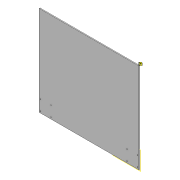
# Autodesk Inventor part: voetensteun
Saved by Autodesk Inventor 2020.3 (Build 243373000, 373)
## iProperties
Created: 2020-09-30
Part Number: voetensteun
Material: Generic
Document SubType Name: Sheet Metal
Designer: Svend
Density: 1 g/cm^3
Appearance: Default
Sheet Metal Rule: Default
Author: Svend
Autodesk Inventor part; units mm, degrees
ref_plane "YZ Plane" through (0, 0, 0) normal (1, 0, 0) x (0, 1, 0)
ref_plane "XZ Plane" through (0, 0, 0) normal (0, 1, 0) x (-1, 0, 0)
ref_plane "XY Plane" through (0, 0, 0) normal (0, 0, 1) x (1, 0, 0)
ref_plane "Work Plane1" through (0, 10, 0) normal (0, 0, 1) x (1, 0, 0)
sketch "Sketch1" plane through (0, 10, 0) normal (0, 0, 1) x (1, 0, 0)
  line L0 (-1, 70.8708) -> (-1, -7.0974) projected
  line L1 (-1, 70.8708) -> (-53.0809, 70.8708) projected
  arc A0 (-53.0809, 70.8708) -> (-59.8755, 68.2079) centre (-53.0809, 60.8708) ccw projected
  line L2 (-59.8755, 68.2079) -> (-118.9152, 13.5337) projected
  line L3 (-1, -7.0974) -> (-454, -7.0974) projected
  circle A1 centre (-53.25, 13.6208) radius 2.067 projected
  circle A2 centre (-53.25, 61.1208) radius 2.067 projected
  circle A3 centre (-5.75, 13.6208) radius 2.067 projected
  circle A4 centre (-5.75, 61.1208) radius 2.067 projected
  circle A5 centre (-401.75, 61.1208) radius 2.067 projected
  circle A6 centre (-449.25, 61.1208) radius 2.067 projected
  circle A7 centre (-401.75, 13.6208) radius 2.067 projected
  circle A8 centre (-449.25, 13.6208) radius 2.067 projected
  line L4 (-454, -7.0974) -> (-454, 70.8708) projected
  line L5 (-1, -7.0974) -> (-454, -7.0974) projected
  arc A9 (-344.754, 14.034) -> (-337.4562, 10.8708) centre (-337.4562, 20.8708) ccw projected
  line L6 (-344.754, 14.034) -> (-395.0366, 67.7076) projected
  arc A10 (-395.0366, 67.7076) -> (-402.3345, 70.8708) centre (-402.3345, 60.8708) ccw projected
  line L7 (-402.3345, 70.8708) -> (-454, 70.8708) projected
  arc A11 (-436.1083, -78.4697) -> (-447.5, -37.6782) centre (-447.5, -59.6646) ccw projected
  line L8 (-18.8917, -78.4697) -> (-436.1083, -78.4697) projected
  arc A12 (-7.5, -37.6782) -> (-18.8917, -78.4697) centre (-7.5, -59.6646) ccw projected
  line L9 (-2, -37.6782) -> (-7.5, -37.6782) projected
  arc A13 (-2, -37.6782) -> (-1, -36.6782) centre (-2, -36.6782) ccw projected
  line L10 (-1, -12.4515) -> (-1, -36.6782) projected
  line L11 (-454, -12.4515) -> (-1, -12.4515) projected
  line L12 (-454, -36.6782) -> (-454, -12.4515) projected
  arc A14 (-454, -36.6782) -> (-453, -37.6782) centre (-453, -36.6782) ccw projected
  line L13 (-447.5, -37.6782) -> (-453, -37.6782) projected
  line L14 (-237.5, -48.429) -> (-237.5, -34.9155) projected
  ellipse E0 centre (-235.5, -34.9155) end of major axis (-237.5, -34.9155) minor radius 1.6892 (-235.5, -33.2263) -> (-237.5, -34.9155) ccw projected
  line L15 (-235.5, -33.2263) -> (-219.5, -33.2263) projected
  ellipse E1 centre (-219.5, -34.9155) end of major axis (-221.5, -34.9155) minor radius 1.6892 (-217.5, -34.9155) -> (-219.5, -33.2263) ccw projected
  line L16 (-217.5, -34.9155) -> (-217.5, -48.429) projected
  ellipse E2 centre (-219.5, -48.429) end of major axis (-217.5, -48.429) minor radius 1.6892 (-219.5, -50.1182) -> (-217.5, -48.429) ccw projected
  line L17 (-219.5, -50.1182) -> (-235.5, -50.1182) projected
  ellipse E3 centre (-235.5, -48.429) end of major axis (-233.5, -48.429) minor radius 1.6892 (-237.5, -48.429) -> (-235.5, -50.1182) ccw projected
  line L18 (-267.5, -48.429) -> (-267.5, -34.9155) projected
  ellipse E4 centre (-265.5, -34.9155) end of major axis (-267.5, -34.9155) minor radius 1.6892 (-265.5, -33.2263) -> (-267.5, -34.9155) ccw projected
  line L19 (-265.5, -33.2263) -> (-249.5, -33.2263) projected
  ellipse E5 centre (-249.5, -34.9155) end of major axis (-251.5, -34.9155) minor radius 1.6892 (-247.5, -34.9155) -> (-249.5, -33.2263) ccw projected
  line L20 (-247.5, -34.9155) -> (-247.5, -48.429) projected
  ellipse E6 centre (-249.5, -48.429) end of major axis (-247.5, -48.429) minor radius 1.6892 (-249.5, -50.1182) -> (-247.5, -48.429) ccw projected
  line L21 (-249.5, -50.1182) -> (-265.5, -50.1182) projected
  ellipse E7 centre (-265.5, -48.429) end of major axis (-263.5, -48.429) minor radius 1.6892 (-267.5, -48.429) -> (-265.5, -50.1182) ccw projected
  line L22 (-205.5, -33.2263) -> (-189.5, -33.2263) projected
  ellipse E8 centre (-189.5, -34.9155) end of major axis (-191.5, -34.9155) minor radius 1.6892 (-187.5, -34.9155) -> (-189.5, -33.2263) ccw projected
  line L23 (-187.5, -34.9155) -> (-187.5, -48.429) projected
  ellipse E9 centre (-189.5, -48.429) end of major axis (-187.5, -48.429) minor radius 1.6892 (-189.5, -50.1182) -> (-187.5, -48.429) ccw projected
  line L24 (-189.5, -50.1182) -> (-205.5, -50.1182) projected
  ellipse E10 centre (-205.5, -48.429) end of major axis (-203.5, -48.429) minor radius 1.6892 (-207.5, -48.429) -> (-205.5, -50.1182) ccw projected
  line L25 (-207.5, -48.429) -> (-207.5, -34.9155) projected
  ellipse E11 centre (-205.5, -34.9155) end of major axis (-207.5, -34.9155) minor radius 1.6892 (-205.5, -33.2263) -> (-207.5, -34.9155) ccw projected
  line L26 (-395, -52.2297) -> (-395, -31.1148) projected
  ellipse E12 centre (-385, -31.1148) end of major axis (-395, -31.1148) minor radius 8.4459 (-385, -22.6689) -> (-395, -31.1148) ccw projected
  line L27 (-385, -22.6689) -> (-310, -22.6689) projected
  ellipse E13 centre (-310, -31.1148) end of major axis (-320, -31.1148) minor radius 8.4459 (-300, -31.1148) -> (-310, -22.6689) ccw projected
  line L28 (-300, -31.1148) -> (-300, -52.2297) projected
  ellipse E14 centre (-310, -52.2297) end of major axis (-300, -52.2297) minor radius 8.4459 (-310, -60.6756) -> (-300, -52.2297) ccw projected
  line L29 (-310, -60.6756) -> (-385, -60.6756) projected
  ellipse E15 centre (-385, -52.2297) end of major axis (-375, -52.2297) minor radius 8.4459 (-395, -52.2297) -> (-385, -60.6756) ccw projected
  line L30 (-145, -22.6689) -> (-70, -22.6689) projected
  ellipse E16 centre (-70, -31.1148) end of major axis (-80, -31.1148) minor radius 8.4459 (-60, -31.1148) -> (-70, -22.6689) ccw projected
  line L31 (-60, -31.1148) -> (-60, -52.2297) projected
  ellipse E17 centre (-70, -52.2297) end of major axis (-60, -52.2297) minor radius 8.4459 (-70, -60.6756) -> (-60, -52.2297) ccw projected
  line L32 (-70, -60.6756) -> (-145, -60.6756) projected
  ellipse E18 centre (-145, -52.2297) end of major axis (-135, -52.2297) minor radius 8.4459 (-155, -52.2297) -> (-145, -60.6756) ccw projected
  line L33 (-155, -52.2297) -> (-155, -31.1148) projected
  ellipse E19 centre (-145, -31.1148) end of major axis (-155, -31.1148) minor radius 8.4459 (-145, -22.6689) -> (-155, -31.1148) ccw projected
  circle A15 centre (-53.25, 13.6208) radius 2.067 projected
  circle A16 centre (-53.25, 61.1208) radius 2.067 projected
  circle A17 centre (-5.75, 13.6208) radius 2.067 projected
  circle A18 centre (-5.75, 61.1208) radius 2.067 projected
  line L34 (-1, 70.8708) -> (-1, -7.0974) projected
  line L35 (-1, 70.8708) -> (-53.0809, 70.8708) projected
  arc A19 (-53.0809, 70.8708) -> (-59.8755, 68.2079) centre (-53.0809, 60.8708) ccw projected
  line L36 (-59.8755, 68.2079) -> (-118.9152, 13.5337) projected
  arc A20 (-125.7098, 10.8708) -> (-118.9152, 13.5337) centre (-125.7098, 20.8708) ccw projected
  line L37 (-125.7098, 10.8708) -> (-337.4562, 10.8708) projected
  circle A21 centre (-449.25, 13.6208) radius 2.067 projected
  circle A22 centre (-401.75, 13.6208) radius 2.067 projected
  circle A23 centre (-449.25, 61.1208) radius 2.067 projected
  circle A24 centre (-401.75, 61.1208) radius 2.067 projected
  line L38 (-454, -7.0974) -> (-454, 70.8708) projected
  arc A25 (-125.7098, 10.8708) -> (-118.9152, 13.5337) centre (-125.7098, 20.8708) ccw projected
  line L39 (-125.7098, 10.8708) -> (-337.4562, 10.8708) projected
  arc A26 (-344.754, 14.034) -> (-337.4562, 10.8708) centre (-337.4562, 20.8708) ccw projected
  line L40 (-344.754, 14.034) -> (-395.0366, 67.7076) projected
  arc A27 (-395.0366, 67.7076) -> (-402.3345, 70.8708) centre (-402.3345, 60.8708) ccw projected
  line L41 (-402.3345, 70.8708) -> (-454, 70.8708) projected
  circle A28 centre (-227.5, 1.8867) radius 4
  line L42 (-227.5, 1.8867) -> (-227.5, -7.0974) construction
  line L43 (-227.5, 1.8867) -> (-227.5, 10.8708) construction
  line L44 (51.5, 217.3708) -> (43.5, 217.3708)
  line L45 (-506.5, 217.3708) -> (-498.5, 217.3708)
  line L46 (-1, -7.0974) -> (-454, -7.0974)
  line L47 (-455, 417.3708) -> (0, 417.3708)
  line L48 (-455, 70.8708) -> (-455, 6.8872) projected
  line L49 (0, -7.0974) -> (0, 70.8708) projected
  line L50 (-455, -7.0974) -> (-455, 417.3708)
  line L51 (0, -7.0974) -> (0, 417.3708)
  line L52 (-1, -7.0974) -> (0, -7.0974)
  line L53 (-454, -7.0974) -> (-455, -7.0974)
  point P0 (0, -10)
  point P1 (-227.5, -33.2263)
  point P2 (0, 70.8708)
  point P3 (-455, 6.8872)
  point P4 (-454, -7.0974)
  dimension "d0" = 8
  dimension "d1" = 200
  constraints: 20 end point, 4 collinear, 4 horizontal, 3 point on line, 2 midpoint, 1 centre point, 1 parallel, 1 vertical alignment, 24 other
  measures "d0" diameter of A28
  measures "d1" distance between parallel lines of L45 L47
extrude "Extrusion1" add sketch "Sketch1" along normal blind 4 contours L1 A0 L2 A20 L37 A9 L6 A10 L7 L4 L53 L50 L48 L47 L51 L49 L52 L0 | L0 L3 L4 L7 A10 L6 A9 L37 A20 L2 A0 L1
sketch "Sketch2" plane through (0, 10, 4) normal (0, 0, 1) x (1, 0, 0)
  line L0 (0, -7.0974) -> (0, 417.3708) projected
  line L1 (0, 417.3708) -> (-455, 417.3708) projected
  line L2 (-455, 417.3708) -> (-455, -7.0974) projected
  line L3 (-455, -7.0974) -> (0, -7.0974) projected
  circle A0 centre (-227.5, 1.8867) radius 4 projected
  circle A1 centre (-449.25, 13.6208) radius 2.067 projected
  circle A2 centre (-53.25, 13.6208) radius 2.067 projected
  circle A3 centre (-53.25, 61.1208) radius 2.067 projected
  circle A4 centre (-5.75, 13.6208) radius 2.067 projected
  circle A5 centre (-5.75, 61.1208) radius 2.067 projected
  circle A6 centre (-401.75, 61.1208) radius 2.067 projected
  circle A7 centre (-449.25, 61.1208) radius 2.067 projected
  circle A8 centre (-401.75, 13.6208) radius 2.067 projected
  line L4 (-455, 417.3708) -> (-455, -7.0974) projected
  line L5 (0, -7.0974) -> (-455, -7.0974)
  line L6 (-455, -7.0974) -> (-455, 5.8867)
  line L7 (-455, 5.8867) -> (0, 5.8867)
  line L8 (0, 5.8867) -> (0, -7.0974)
  point P0 (0, -10)
  constraints: 8 end point, 2 parallel, 1 horizontal, 1 perpendicular, 1 point on line, 1 tangent
extrude "Cut1" cut sketch "Sketch2" against normal up to next contours L3 L2 L7 L0
equation "\"d5\" = Thickness"
equation "\"BendRadius\" = Thickness"
equation "\"BendReliefWidth\" = Thickness"
equation "\"BendReliefDepth\" = 0.5 * Thickness"
equation "\"CornerReliefSize\" = 4 * Thickness"
equation "\"MinimumRemnant\" = 2 * Thickness"
equation "\"TransitionRadius\" = BendRadius"
equation "\"JacobiRadiusSize\" = Thickness"
equation "\"GapSize\" = Thickness"
equation "\"d4\" = Thickness"
equation "\"Thickness\" = 0.5"
body "Solid1"
